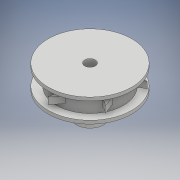
# Autodesk Inventor part: intermediateSpindle
Saved by Autodesk Inventor 2018 (Build 220112000, 112)
## iProperties
Created: 2017-10-22
Part Number: intermediateSpindle
Material: Generic
Document SubType Name: Modeling
Designer: Prakash
Density: 1 g/cm^3
Appearance: Default
Author: Prakash
Autodesk Inventor part; units mm, degrees
ref_plane "XZ Plane" through (0, 0, 0) normal (0, 1, 0) x (-1, 0, 0)
ref_plane "XY Plane" through (0, 0, 0) normal (0, 0, 1) x (1, 0, 0)
sketch "Sketch1" plane through (0, 0, 0) normal (0, 0, 1) x (1, 0, 0)
  circle A0 centre (0, 0) radius 20
  circle A1 centre (0, 0) radius 25
  circle A2 centre (0, 0) radius 3.175
  circle A3 centre (0, 0) radius 8.175
  dimension "d18" = 6.35
  dimension "d19" = 16.35
  dimension "d40" = 40
  dimension "d41" = 5
  constraints: 4 centre point, 4 coincident
  measures "d18" diameter of A2
  measures "d19" diameter of A3
  measures "d40" diameter of A0
  measures "d41" radial gap between concentric circles of A1 A0
extrude "Extrusion1" add sketch "Sketch1" along normal blind 14 contours A0 | A2 | A3
extrude "Extrusion2" add sketch "Sketch1" along normal blind 2 contours A1
sketch "Sketch2" plane through (0, 0, 14) normal (0, 0, 1) x (1, 0, 0)
  circle A0 centre (0, 0) radius 20 projected
  circle A1 centre (0, 0) radius 25 projected
extrude "Extrusion3" add sketch "Sketch2" against normal blind 2
ref_plane "Work Plane1" through (0, 0, 7) normal (0, 0, -1) x (-1, 0, 0)
extrude "Extrusion5" cut sketch "Sketch1" along normal up to surface (14 mm away) contours A2
extrude "Extrusion6" add sketch "Sketch1" against normal blind 14 contours A3
ref_plane "Work Plane2" through (8.175, 0, 0) normal (1, 0, 0) x (0, 1, 0)
sketch "Sketch4" plane through (8.175, 0, 0) normal (1, 0, 0) x (0, 1, 0)
  line L0 (8.175, 0) -> (-8.175, 0) projected
  line L1 (-8.175, -14) -> (8.175, -14) projected
  line L2 (0, 0) -> (0, -14)
  line L3 (-2.3094, -11) -> (-4.6188, -7)
  line L4 (-4.6188, -7) -> (-2.3094, -3)
  line L5 (-2.3094, -3) -> (2.3094, -3)
  line L6 (2.3094, -3) -> (4.6188, -7)
  line L7 (4.6188, -7) -> (2.3094, -11)
  line L8 (2.3094, -11) -> (-2.3094, -11)
  point P0 (0, -7)
  point P1 (0, -11)
  dimension "d24" = 8
  constraints: 14 end point, 3 midpoint, 1 point on line, 13 other
  measures "d24" distance between parallel lines of L4 L7
hole "Hole1" at (8.175, 0, -7) direction (-1, 0, 0) diameter 3 end up to face face through (0, 0, 0) facing (0, 0, 1) round with radius 3.175 far side yes
extrude "Extrusion7" cut sketch "Sketch4" against normal blind 3.175
sketch "Sketch9" plane through (0, 0, 7) normal (0, 0, -1) x (-1, 0, 0)
  circle A0 centre (0, 0) radius 20 projected
  line L0 (0, -20) -> (0, -25) construction
  circle A1 centre (0, 0) radius 25 projected
  arc A2 (0, -20) -> (0, -25) centre (7.5993, -22.5) ccw
  line L1 (0, -25) -> (-4.6567, -19.4503)
  circle A3 centre (0, 0) radius 20
  line L2 (17.3205, -10) -> (21.6506, -12.5) construction
  line L3 (21.6506, -12.5) -> (14.5161, -13.758)
  arc A4 (17.3205, -10) -> (21.6506, -12.5) centre (23.2852, -4.6688) ccw
  line L4 (17.3205, 10) -> (21.6506, 12.5) construction
  line L5 (21.6506, 12.5) -> (19.1728, 5.6923)
  arc A5 (17.3205, 10) -> (21.6506, 12.5) centre (15.6859, 17.8312) ccw
  line L6 (0, 20) -> (0, 25) construction
  line L7 (0, 25) -> (4.6567, 19.4503)
  arc A6 (0, 20) -> (0, 25) centre (-7.5993, 22.5) ccw
  line L8 (-17.3205, 10) -> (-21.6506, 12.5) construction
  line L9 (-21.6506, 12.5) -> (-14.5161, 13.758)
  arc A7 (-17.3205, 10) -> (-21.6506, 12.5) centre (-23.2852, 4.6688) ccw
  line L10 (-17.3205, -10) -> (-21.6506, -12.5) construction
  line L11 (-21.6506, -12.5) -> (-19.1728, -5.6923)
  arc A8 (-17.3205, -10) -> (-21.6506, -12.5) centre (-15.6859, -17.8312) ccw
  point P0 (0, -22.5)
  point P1 (19.4856, -11.25)
  point P2 (19.4856, 11.25)
  point P3 (0, 22.5)
  point P4 (-19.4856, 11.25)
  point P5 (-19.4856, -11.25)
  dimension "d58" = 8
  dimension "d59" = 40
  dimension "d62" = 360
  constraints: 24 end point, 12 point on circle, 7 centre point, 2 vertical, 1 coincident, 1 midpoint, 1 vertical alignment, 64 other
  measures "d58" radius of A2
  measures "d59" angle of L1 L0
extrude "Extrusion9" add sketch "Sketch9" along normal mid plane 4 contours A0 A5 L5 | A4 L3 A0 | A0 A6 L7 | A2 L1 A0 | L9 A0 A7 | L11 A0 A8
body "Solid1"
